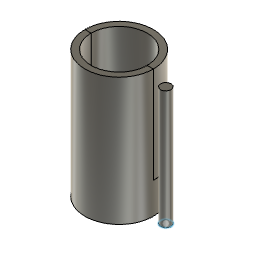
capsule_biopsy_mold v4 (Autodesk Fusion 360 design; units mm, degrees)
Autodesk Fusion 360 part; units mm, degrees
sketch "Sketch4" plane through (0, 0, 0) normal (0, 0, 1) x (1, 0, 0)
  circle A0 centre (0, 0) radius 55
  circle A1 centre (0, 0) radius 45
  dimension "d11" = 110
  dimension "d12" = 90
  constraint coincident A0.centre A1.centre
  constraint concentric A0 A1
  measures "d11" diameter of A0
  measures "d12" diameter of A1
extrude "Extrude2" add sketch "Sketch4" along normal blind 155 makes body 1
move_body "Move1" bodies 1 to x (1, 0, 0) y (0, 1, 0) z (0, 0, 1) at (0, 0, 50)
sketch "Sketch5" plane through (0, 0, 0) normal (0, 0, 1) x (1, 0, 0)
  circle A0 centre (0, 0) radius 55
  dimension "d15" = 110
  constraint coincident A0.centre origin
  measures "d15" diameter of A0
extrude "Extrude3" add sketch "Sketch5" along normal blind 50 bodies 1
sketch "Sketch6" plane through (0, 0, 50) normal (0, 0, 1) x (-1, 0, 0)
  circle A0 centre (0, 0) radius 45
  circle A1 centre (0, 0) radius 8.337
  dimension "d18" = 16.674
  constraint coincident A0.centre A1.centre
  measures "d18" diameter of A1
extrude "Extrude4" cut sketch "Sketch6" against normal blind 25.4 contours A1 bodies 1
split_face "SplitFace1" 1 faces at (51.2944, -4.9681, 205) by bodies 1 on bodies 1
sketch "Sketch7" plane through (0, 0, 0) normal (1, 0, 0) x (0, 1, 0)
  line L0 (-78.7313, 243.4439) -> (103.7817, 243.4439)
  line L1 (103.7817, 243.4439) -> (103.7817, 50)
  line L2 (103.7817, 50) -> (-78.7313, 50)
  line L3 (-78.7313, 50) -> (-78.7313, 243.4439)
  line L4 (55, 0) -> (-55, 0)
  dimension "d22" = 50
  constraint horizontal L0
  constraint vertical L1
  constraint horizontal L2
  constraint vertical L3
  measures "d22" distance of L2 L4
split "Split1" by curves path "Sketch7" along L3 L0 L1 L2 bodies 1 makes body 2 at (54.7267, -5.4762, 16.6667)
split "Split2" by plane through (0, 0, 0) normal (0, 1, 0) bodies 1 makes body 3 at (54.7267, 5.4762, 101.6667)
combine "Combine1" operation add target body 1 tool bodies 2
sketch "Sketch8" plane through (0, 0, 0) normal (0, 0, 1) x (1, 0, 0)
  circle A0 centre (75, 0) radius 8.337
  dimension "d25" = 16.674
  measures "d25" diameter of A0
extrude "Extrude6" add sketch "Sketch8" along normal blind 190.4 separate body makes body 4
equation "esophagus_diam = 16.674 mm"
equation "neck_rad = 45 mm"
equation "d11 = neck_rad * 2 + 20 mm"
equation "d12 = neck_rad * 2"
equation "d15 = neck_rad * 2 + 20 mm"
equation "d18 = esophagus_diam"
equation "d22 = ground_offset"
equation "rod_insert = 25.4 mm"
equation "ground_offset = 50 mm"
equation "d25 = esophagus_diam"
equation "base_to_top = 165 mm"
equation "rod_length = base_to_top + 25.4 mm"
equation "d30 = rod_length"
named bodies: "Mold Base", "Mold Wall", "Esophagus Negative"
